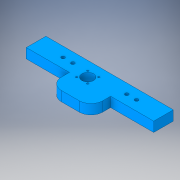
# Autodesk Inventor part: GripperM otorBlock
Saved by Autodesk Inventor 2019 (Build 230136000, 136)
## iProperties
Created: 2019-10-02
Part Number: GripperM otorBlock
Material: Generic
Document SubType Name: Modeling
Designer: james
Density: 1 g/cm^3
Appearance: Default(2)
Author: james
Autodesk Inventor part; units mm, degrees
ref_plane "YZ Plane" through (0, 0, 0) normal (1, 0, 0) x (0, 1, 0)
ref_plane "XZ Plane" through (0, 0, 0) normal (0, 1, 0) x (-1, 0, 0)
ref_plane "XY Plane" through (0, 0, 0) normal (0, 0, 1) x (1, 0, 0)
sketch "Sketch1" plane through (0, 0, 0) normal (1, 0, 0) x (0, 1, 0)
  line L0 (11.2985, 26.2091) -> (-1.4015, 26.2091)
  line L1 (-1.4015, 26.2091) -> (-1.4015, -24.5909)
  line L2 (-1.4015, -24.5909) -> (11.2985, -24.5909)
  line L3 (11.2985, -24.5909) -> (11.2985, 26.2091)
  point P0 (0, 0)
  dimension "d0" = 50.8
  dimension "d1" = 12.7
  constraints: 8 end point, 2 parallel, 1 horizontal, 1 perpendicular
  measures "d0" distance of L2.end L0.start
  measures "d1" distance of L0.start L0.end
extrude "Extrusion1" add sketch "Sketch1" along normal blind 165.1
sketch "Sketch2" plane through (0, 11.2985, 26.2091) normal (0, 1, 0) x (1, 0, 0)
  circle A0 centre (73.025, 32.004) radius 12.7
  circle A1 centre (92.075, 32.004) radius 12.7
  line L0 (0, 50.8) -> (0, 0) projected
  line L1 (0, 50.8) -> (165.1, 50.8) projected
  point P0 (0, 26.2091)
  point P1 (65.8495, 39.1795)
  point P2 (80.2005, 39.1795)
  point P3 (80.2005, 24.8285)
  point P4 (65.8495, 24.8285)
  dimension "d4" = 25.4
  dimension "d5" = 25.4
  dimension "d6" = 0
  dimension "d7" = 19.05
  dimension "d8" = 73.025
  dimension "d9" = 18.796
  dimension "d46" = 0
  dimension "d47" = 0
  dimension "d48" = 0
  dimension "d49" = 0
  dimension "d50" = 14.351
  dimension "d51" = 14.351
  dimension "d52" = 7.1755
  dimension "d53" = 7.1755
  constraints: 2 centre point
  measures "d4" diameter of A0
  measures "d5" diameter of A1
  measures "d6" vertical distance of A0.centre A1.centre
  measures "d7" distance of A0.centre A1.centre
  measures "d8" distance from line of L0 A0.centre
  measures "d9" distance from line of L1 A0.centre
  measures "d46" horizontal distance of point (65.85, 24.828) point (65.85, 39.179)
  measures "d47" horizontal distance of point (80.201, 39.179) point (80.201, 24.828)
  measures "d48" vertical distance of point (65.85, 24.828) point (80.201, 24.828)
  measures "d49" vertical distance of point (65.85, 39.179) point (80.201, 39.179)
  measures "d50" distance of point (80.201, 39.179) point (65.85, 39.179)
  measures "d51" distance of point (65.85, 24.828) point (65.85, 39.179)
  measures "d52" horizontal distance of point (65.85, 39.179) A0.centre
  measures "d53" horizontal distance of A0.centre point (65.85, 24.828)
sketch "Sketch8" plane through (0, 11.2985, 26.2091) normal (0, 1, 0) x (1, 0, 0)
  line L0 (-37.599, -14.8006) -> (55.88, -14.8006)
  line L1 (55.88, -14.8006) -> (55.88, 38.1)
  line L2 (55.88, 38.1) -> (-37.599, 38.1)
  line L3 (-37.599, 38.1) -> (-37.599, -14.8006)
  line L4 (109.22, -16.386) -> (193.9952, -16.386)
  line L5 (193.9952, -16.386) -> (193.9952, 38.1)
  line L6 (193.9952, 38.1) -> (109.22, 38.1)
  line L7 (109.22, 38.1) -> (109.22, -16.386)
  line L8 (0, 50.8) -> (165.1, 50.8) projected
  line L9 (0, 50.8) -> (0, 0) projected
  line L10 (165.1, 50.8) -> (165.1, 0) projected
  point P0 (0, 26.2091)
  dimension "d36" = 12.7
  dimension "d37" = 55.88
  dimension "d38" = 12.7
  dimension "d39" = 55.88
  constraints: 16 end point, 4 parallel, 2 horizontal, 2 perpendicular
  measures "d36" distance between parallel lines of L2 L8
  measures "d37" distance between parallel lines of L9 L1
  measures "d38" distance between parallel lines of L8 L6
  measures "d39" distance between parallel lines of L10 L7
extrude "Extrusion8" cut sketch "Sketch8" against normal blind 76.2
fillet "Fillet1" radius 15.24 1 edges at (109.22, 4.9485, 26.2091)
fillet "Fillet2" radius 15.24 1 edges at (55.88, 4.9485, 26.2091)
hole "Hole1" at (65.8495, 11.2985, -12.9704) at (80.2005, 11.2985, -12.9704) at (80.2005, 11.2985, 1.3806) at (65.8495, 11.2985, 1.3806) direction (0, -1, 0) diameter 2.4384 end through all clearance for "Flat Head Machine Screw (82)" size "#2" standard "Ansi Unified Screw Threads"
sketch "Sketch10" plane through (0, 11.2985, -24.5909) normal (0, 1, 0) x (1, 0, 0)
  circle A0 centre (80.2005, -25.9715) radius 1.2192 projected
  circle A1 centre (65.8495, -11.6205) radius 1.2192 projected
  circle A2 centre (65.8495, -25.9715) radius 1.2192 projected
  circle A3 centre (80.2005, -11.6205) radius 1.2192 projected
  line L0 (80.2005, -11.6205) -> (65.8495, -25.9715)
  line L1 (65.8495, -11.6205) -> (80.2005, -25.9715)
  point P0 (0, -24.5909)
  point P1 (73.025, -18.796)
  dimension "d61" = 7.1755
  dimension "d62" = 7.1755
  constraints: 4 end point
  measures "d61" horizontal distance of point (73.025, -18.796) L1.start
  measures "d62" horizontal distance of point (73.025, -18.796) L0.start
hole "Hole2" at (73.025, 11.2985, -5.7949) direction (0, -1, 0) diameter 15.24 end through all
sketch "Sketch11" plane through (0, 11.2985, -11.8909) normal (0, 0, 1) x (1, 0, 0)
  line L0 (55.88, 0) -> (0, 0)
  line L1 (0, 0) -> (0, -12.7)
  line L2 (0, -12.7) -> (55.88, -12.7)
  line L3 (55.88, -12.7) -> (55.88, 0)
  line L4 (0, -12.7) -> (0, 0) projected
  line L5 (55.88, 0) -> (55.88, -12.7) projected
  line L6 (0, 0) -> (55.88, 0) projected
  line L7 (55.88, -12.7) -> (0, -12.7) projected
  point P0 (0, -11.2985)
  dimension "d70" = 0
  dimension "d71" = 0
  dimension "d72" = 0
  dimension "d73" = 0
  constraints: 8 end point, 2 parallel, 1 horizontal, 1 perpendicular
  measures "d70" distance between parallel lines of L4 L1
  measures "d71" distance between parallel lines of L5 L3
  measures "d72" distance between parallel lines of L6 L0
  measures "d73" distance between parallel lines of L7 L2
extrude "Extrusion9" add sketch "Sketch11" along normal blind 12.7
sketch "Sketch12" plane through (109.22, 11.2985, -11.8909) normal (0, 0, 1) x (1, 0, 0)
  line L0 (0, 0) -> (55.88, 0)
  line L1 (55.88, 0) -> (55.88, -12.7)
  line L2 (55.88, -12.7) -> (0, -12.7)
  line L3 (0, -12.7) -> (0, 0)
  line L4 (55.88, 0) -> (55.88, -12.7) projected
  line L5 (0, 0) -> (55.88, 0) projected
  line L6 (55.88, -12.7) -> (0, -12.7) projected
  line L7 (0, -12.7) -> (0, 0) projected
  point P0 (-109.22, -11.2985)
  dimension "d76" = 0
  dimension "d77" = 0
  dimension "d78" = 0
  dimension "d79" = 0
  constraints: 8 end point, 2 parallel, 1 horizontal, 1 perpendicular
  measures "d76" distance between parallel lines of L4 L1
  measures "d77" distance between parallel lines of L5 L0
  measures "d78" distance between parallel lines of L6 L2
  measures "d79" distance between parallel lines of L7 L3
extrude "Extrusion10" add sketch "Sketch12" along normal blind 12.7
sketch "Sketch13" plane through (0, 11.2985, -24.5909) normal (0, 1, 0) x (1, 0, 0)
  line L0 (55.88, -25.4) -> (55.88, -35.56) projected
  line L1 (0, 0) -> (165.1, 0) projected
  line L2 (109.22, -35.56) -> (109.22, -25.4) projected
  point P0 (0, -24.5909)
  point P1 (47.625, -12.7)
  point P2 (34.925, -12.7)
  point P3 (117.475, -12.7)
  point P4 (130.175, -12.7)
  dimension "d82" = 20.955
  dimension "d83" = 8.255
  dimension "d84" = 12.7
  dimension "d85" = 12.7
  dimension "d86" = 8.255
  dimension "d87" = 20.955
  dimension "d88" = 12.7
  dimension "d89" = 12.7
  measures "d82" distance from line of L0 point (34.925, -12.7)
  measures "d83" distance from line of L0 point (47.625, -12.7)
  measures "d84" distance from line of L1 point (47.625, -12.7)
  measures "d85" distance from line of L1 point (34.925, -12.7)
  measures "d86" distance from line of L2 point (117.475, -12.7)
  measures "d87" distance from line of L2 point (130.175, -12.7)
  measures "d88" distance from line of L1 point (117.475, -12.7)
  measures "d89" distance from line of L1 point (130.175, -12.7)
hole "Hole3" at (47.625, 11.2985, -11.8909) at (34.925, 11.2985, -11.8909) at (117.475, 11.2985, -11.8909) at (130.175, 11.2985, -11.8909) direction (0, -1, 0) diameter 4.4958 depth 25.4 tip angle 118.188 clearance for "Flat Head Machine Screw (82)" size "#8" standard "Ansi Unified Screw Threads"
body "Solid1"
